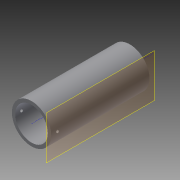
# Autodesk Inventor part: cylinder
Saved by Autodesk Inventor 2015 SP2 (Build 190223200, 223)
## iProperties
Created: 2016-03-07
Part Number: cylinder
Material: Generic
Document SubType Name: Modeling
Designer: marc
Density: 1 g/cm^3
Appearance: Default
Author: marc
Autodesk Inventor part; units mm, degrees
ref_plane "XZ Plane" through (0, 0, 0) normal (0, 1, 0) x (-1, 0, 0)
ref_plane "XY Plane" through (0, 0, 0) normal (0, 0, 1) x (1, 0, 0)
sketch "Sketch1" plane through (0, 0, 0) normal (0, 1, 0) x (-1, 0, 0)
  circle A0 centre (0, 0) radius 25
  circle A1 centre (0, 0) radius 30
  dimension "ID" = 50
  dimension "thickness" = 5
  constraints: 2 centre point, 2 coincident
  measures "ID" diameter of A0
  measures "thickness" radial gap between concentric circles of A1 A0
extrude "Extrusion1" add sketch "Sketch1" along normal blind 150
ref_plane "Work Plane1" through (30, 0, 0) normal (1, 0, 0) x (0, 1, 0)
sketch "Sketch2" plane through (30, 0, 0) normal (1, 0, 0) x (0, 1, 0)
  line L0 (0, 0) -> (214.2625, 0) construction
  line L1 (0, 30) -> (0, -30) projected
  point P0 (10, 0)
  dimension "holeOffset" = 10
  constraints: 2 end point, 1 horizontal, 1 point on line
  measures "holeOffset" distance from line of point (10, 0) L1
hole "Hole1" at (30, 10, 0) direction (-1, 0, 0) diameter 4.5 end through all clearance for "Socket Head Cap Screw ISO 4762" size "M4" standard "ISO"
sketch "Sketch3" plane through (0, 0, 0) normal (1, 0, 0) x (0, 1, 0)
  line L0 (0, 0) -> (185.9449, 0) construction
  constraints: 2 end point, 1 horizontal
body "Solid1"
